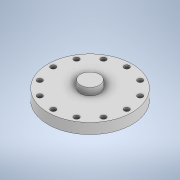
# Autodesk Inventor part: magnet bottom
Saved by Autodesk Inventor 2021 (Build 250183000, 183)
## iProperties
Created: 2022-10-28
Part Number: magnet bottom
Material: Generic
Document SubType Name: Modeling
Designer: warre
Density: 1 g/cm^3
Appearance: Default
Author: warre
Autodesk Inventor part; units mm, degrees
ref_plane "YZ Plane" through (0, 0, 0) normal (1, 0, 0) x (0, 1, 0)
ref_plane "XZ Plane" through (0, 0, 0) normal (0, 1, 0) x (-1, 0, 0)
ref_plane "XY Plane" through (0, 0, 0) normal (0, 0, 1) x (1, 0, 0)
sketch "Sketch1" plane through (0, 0, 0) normal (0, 1, 0) x (-1, 0, 0)
  circle A0 centre (0, 0) radius 40
  line L0 (0, 40) -> (40, 40) construction
  line L1 (0, 0) -> (0, 7.8266) construction
  line L2 (0, 0) -> (7.0888, 0) construction
  dimension "d0" = 80
  constraints: 6 end point, 2 coincident, 2 horizontal, 1 vertical, 1 vertical alignment, 2 other
extrude "Extrusion1" add sketch "Sketch1" along normal blind 10
sketch "Sketch2" plane through (0, 10, 0) normal (0, 1, 0) x (1, 0, 0)
  circle A0 centre (0, 0) radius 40 projected
  line L0 (0, -40) -> (-40, -40) construction
  line L1 (0, 0) -> (0, 3.1787) construction
  line L2 (0, 0) -> (-7.099, 0) construction
  line L3 (0, 0) -> (-40, -40)
  line L4 (0, 0) -> (40, -40)
  line L5 (0, 0) -> (-40, 40)
  line L6 (0, 0) -> (40, 40)
  circle A1 centre (0, 0) radius 40 construction
  line L7 (-28.2843, -28.2843) -> (-24.7487, -24.7487) construction
  circle A2 centre (0, 0) radius 35 construction
  circle A3 centre (-35, 0) radius 2.5
  circle A4 centre (-30.3109, -17.5) radius 2.5
  circle A5 centre (-17.5, -30.3109) radius 2.5
  circle A6 centre (0, -35) radius 2.5
  circle A7 centre (17.5, -30.3109) radius 2.5
  circle A8 centre (30.3109, -17.5) radius 2.5
  circle A9 centre (35, 0) radius 2.5
  circle A10 centre (30.3109, 17.5) radius 2.5
  circle A11 centre (17.5, 30.3109) radius 2.5
  circle A12 centre (0, 35) radius 2.5
  circle A13 centre (-17.5, 30.3109) radius 2.5
  circle A14 centre (-30.3109, 17.5) radius 2.5
  dimension "d4" = 5
  dimension "d5" = 5
  dimension "d8" = 360
  constraints: 16 end point, 13 centre point, 3 point on circle, 3 symmetric about line, 2 horizontal, 2 point on line, 1 coincident, 1 vertical, 1 vertical alignment, 26 other
  measures "d4" distance of L7.start L7.end
  measures "d5" diameter of A3
extrude "Extrusion2" cut sketch "Sketch2" against normal through all contours A3 | A4 | A5 | A6 | A7 | A8 | A9 | A10 | A11 | A12 | A13 | A14
sketch "Sketch3" plane through (0, 0, 0) normal (0, -1, 0) x (1, 0, 0)
  point P0 (0, 0)
sketch "Sketch4" plane through (0, 10, 0) normal (0, 1, 0) x (1, 0, 0)
  circle A0 centre (0, 0) radius 9
  dimension "d12" = 18
  constraints: 1 centre point, 1 coincident
  measures "d12" diameter of A0
extrude "Extrusion3" add sketch "Sketch4" along normal blind 7
body "Solid1"
